Autodesk Inventor part; units mm, degrees
(part 2 of 2)
sketch "Sketch47" plane through (0, 0, 0) normal (0, 0, -1) x (-1, 0, 0)
  arc A0 (-24.47, 4.531) -> (-25.255, 6.4154) centre (-25.8772, 5.0505) ccw projected
  arc A1 (-27.3913, -0.5289) -> (-24.47, 4.531) centre (-29.4449, 4.03) ccw projected
  arc A2 (-29.4158, -0.7913) -> (-27.3913, -0.5289) centre (-28.5449, 0.43) ccw projected
  arc A3 (-29.4158, -0.7913) -> (-29.4739, -0.7913) centre (-29.4449, -0.832) ccw projected
  arc A4 (-31.4984, -0.5289) -> (-29.4739, -0.7913) centre (-30.3449, 0.43) ccw projected
  arc A5 (-34.4197, 4.531) -> (-31.4984, -0.5289) centre (-29.4449, 4.03) ccw projected
  arc A6 (-33.6347, 6.4154) -> (-34.4197, 4.531) centre (-33.0126, 5.0505) ccw projected
  arc A7 (-33.6347, 6.4154) -> (-33.6057, 6.4657) centre (-33.6554, 6.4609) ccw projected
  arc A8 (-32.3662, 8.0878) -> (-33.6057, 6.4657) centre (-32.1126, 6.6094) ccw projected
  arc A9 (-26.5236, 8.0878) -> (-32.3662, 8.0878) centre (-29.4449, 4.03) ccw projected
  arc A10 (-25.2841, 6.4657) -> (-26.5236, 8.0878) centre (-26.7772, 6.6094) ccw projected
  arc A11 (-25.2841, 6.4657) -> (-25.255, 6.4154) centre (-25.2343, 6.4609) ccw projected
  arc A12 (29.4739, -0.7913) -> (31.4984, -0.5289) centre (30.3449, 0.43) ccw projected
  arc A13 (29.4739, -0.7913) -> (29.4158, -0.7913) centre (29.4449, -0.832) ccw projected
  arc A14 (27.3913, -0.5289) -> (29.4158, -0.7913) centre (28.5449, 0.43) ccw projected
  arc A15 (24.47, 4.531) -> (27.3913, -0.5289) centre (29.4449, 4.03) ccw projected
  arc A16 (25.255, 6.4154) -> (24.47, 4.531) centre (25.8772, 5.0505) ccw projected
  arc A17 (25.255, 6.4154) -> (25.2841, 6.4657) centre (25.2343, 6.4609) ccw projected
  arc A18 (26.5236, 8.0878) -> (25.2841, 6.4657) centre (26.7772, 6.6094) ccw projected
  arc A19 (32.3662, 8.0878) -> (26.5236, 8.0878) centre (29.4449, 4.03) ccw projected
  arc A20 (33.6057, 6.4657) -> (32.3662, 8.0878) centre (32.1126, 6.6094) ccw projected
  arc A21 (33.6057, 6.4657) -> (33.6347, 6.4154) centre (33.6554, 6.4609) ccw projected
  arc A22 (34.4197, 4.531) -> (33.6347, 6.4154) centre (33.0126, 5.0505) ccw projected
  arc A23 (31.4984, -0.5289) -> (34.4197, 4.531) centre (29.4449, 4.03) ccw projected
  arc A24 (25.2841, -32.4058) -> (26.5236, -34.0279) centre (26.7772, -32.5495) ccw projected
  arc A25 (25.2841, -32.4058) -> (25.255, -32.3555) centre (25.2343, -32.401) ccw projected
  arc A26 (24.47, -30.4711) -> (25.255, -32.3555) centre (25.8772, -30.9906) ccw projected
  arc A27 (27.3913, -25.4112) -> (24.47, -30.4711) centre (29.4449, -29.97) ccw projected
  arc A28 (29.4158, -25.1488) -> (27.3913, -25.4112) centre (28.5449, -26.37) ccw projected
  arc A29 (29.4158, -25.1488) -> (29.4739, -25.1488) centre (29.4449, -25.1081) ccw projected
  arc A30 (31.4984, -25.4112) -> (29.4739, -25.1488) centre (30.3449, -26.37) ccw projected
  arc A31 (34.4197, -30.4711) -> (31.4984, -25.4112) centre (29.4449, -29.97) ccw projected
  arc A32 (33.6347, -32.3555) -> (34.4197, -30.4711) centre (33.0126, -30.9906) ccw projected
  arc A33 (33.6347, -32.3555) -> (33.6057, -32.4058) centre (33.6554, -32.401) ccw projected
  arc A34 (32.3662, -34.0279) -> (33.6057, -32.4058) centre (32.1126, -32.5495) ccw projected
  arc A35 (26.5236, -34.0279) -> (32.3662, -34.0279) centre (29.4449, -29.97) ccw projected
  arc A36 (-11.2583, -6.47) -> (-8.6603, -7.97) centre (-8.6603, -4.97) ccw projected
  line L0 (-11.2583, -6.47) -> (-15.6081, 1.0639) projected
  arc A37 (-15.6081, 1.0639) -> (-20.4883, 4.5367) centre (-21.3982, -1.9073) ccw projected
  arc A38 (-22.8817, 6.4641) -> (-20.4883, 4.5367) centre (-20.0689, 7.5073) ccw projected
  arc A39 (-22.8817, 6.4641) -> (-23.5653, 7.8287) centre (-29.4449, 4.03) ccw projected
  arc A40 (-22.5454, 12.0548) -> (-23.5653, 7.8287) centre (-21.0454, 9.4567) ccw projected
  line L1 (-22.5454, 12.0548) -> (-10.3994, 19.0673) projected
  arc A41 (-6.2296, 17.8374) -> (-10.3994, 19.0673) centre (-8.8994, 16.4692) ccw projected
  arc A42 (-6.2296, 17.8374) -> (-5.3856, 16.5583) centre (0, 21.03) ccw projected
  arc A43 (-4.9109, 13.5211) -> (-5.3856, 16.5583) centre (-7.6937, 14.6419) ccw projected
  arc A44 (-4.9109, 13.5211) -> (-4.4941, 7.8139) centre (1.1185, 11.0927) ccw projected
  line L2 (-4.4941, 7.8139) -> (0.2887, -0.47) projected
  arc A45 (-4.0415, -7.97) -> (0.2887, -0.47) centre (-4.0415, -2.97) ccw projected
  line L3 (-4.0415, -7.97) -> (-8.6603, -7.97) projected
  line L4 (8.9748, -38.4253) -> (8.0248, -40.0706) projected
  arc A46 (3.7987, -41.0905) -> (8.0248, -40.0706) centre (5.4268, -38.5706) ccw projected
  arc A47 (3.7987, -41.0905) -> (0.7829, -40.014) centre (0, -46.97) ccw projected
  arc A48 (-1.4796, -35.5328) -> (0.7829, -40.014) centre (1.1185, -37.0328) ccw projected
  line L5 (-1.4796, -35.5328) -> (5.4642, -23.5057) projected
  arc A49 (12.4713, -23.6489) -> (5.4642, -23.5057) centre (8.9283, -25.5057) ccw projected
  arc A50 (12.4713, -23.6489) -> (15.6795, -27.0233) centre (20, -19.7033) ccw projected
  arc A51 (14.507, -34.3744) -> (15.6795, -27.0233) centre (13.6463, -30.4681) ccw projected
  arc A52 (14.507, -34.3744) -> (8.9748, -38.4253) centre (16.336, -42.6753) ccw projected
  arc A53 (-25.9281, -2.0225) -> (-23.8122, -0.1261) centre (-29.4449, 4.03) ccw projected
  arc A54 (-18.8001, -0.4073) -> (-23.8122, -0.1261) centre (-21.3982, -1.9073) ccw projected
  line L6 (-18.8001, -0.4073) -> (-15.1554, -6.72) projected
  arc A55 (-17.7535, -11.22) -> (-15.1554, -6.72) centre (-17.7535, -8.22) ccw projected
  line L7 (-17.7535, -11.22) -> (-20.7176, -11.22) projected
  arc A56 (-23.3157, -9.72) -> (-20.7176, -11.22) centre (-20.7176, -8.22) ccw projected
  arc A57 (-23.3157, -9.72) -> (-25.8495, -7.2544) centre (-28.9449, -12.97) ccw projected
  arc A58 (-25.9281, -2.0225) -> (-25.8495, -7.2544) centre (-24.4209, -4.6164) ccw projected
  arc A59 (-20.7176, -14.72) -> (-23.3157, -16.22) centre (-20.7176, -17.72) ccw projected
  line L8 (-20.7176, -14.72) -> (-17.7535, -14.72) projected
  arc A60 (-15.1554, -19.22) -> (-17.7535, -14.72) centre (-17.7535, -17.72) ccw projected
  line L9 (-15.1554, -19.22) -> (-18.8001, -25.5328) projected
  arc A61 (-23.8122, -25.814) -> (-18.8001, -25.5328) centre (-21.3982, -24.0328) ccw projected
  arc A62 (-23.8122, -25.814) -> (-25.9281, -23.9176) centre (-29.4449, -29.97) ccw projected
  arc A63 (-25.8495, -18.6857) -> (-25.9281, -23.9176) centre (-24.4209, -21.3237) ccw projected
  arc A64 (-25.8495, -18.6857) -> (-23.3157, -16.22) centre (-28.9449, -12.97) ccw projected
  arc A65 (15.6795, 1.0833) -> (14.507, 8.4344) centre (13.6463, 4.5281) ccw projected
  arc A66 (15.6795, 1.0833) -> (12.4713, -2.2911) centre (20, -6.2367) ccw projected
  arc A67 (5.4642, -2.4343) -> (12.4713, -2.2911) centre (8.9283, -0.4343) ccw projected
  line L10 (5.4642, -2.4343) -> (-1.4796, 9.5927) projected
  arc A68 (0.7829, 14.0739) -> (-1.4796, 9.5927) centre (1.1185, 11.0927) ccw projected
  arc A69 (0.7829, 14.0739) -> (3.7987, 15.1504) centre (0, 21.03) ccw projected
  arc A70 (8.0248, 14.1305) -> (3.7987, 15.1504) centre (5.4268, 12.6305) ccw projected
  line L11 (8.0248, 14.1305) -> (8.9747, 12.4853) projected
  arc A71 (8.9747, 12.4853) -> (14.507, 8.4344) centre (16.336, 16.7353) ccw projected
  arc A72 (23.6453, -24.7033) -> (28.6453, -19.7033) centre (23.6453, -19.7033) ccw projected
  line L12 (23.6453, -24.7033) -> (20, -24.7033) projected
  arc A73 (15, -19.7033) -> (20, -24.7033) centre (20, -19.7033) ccw projected
  line L13 (15, -19.7033) -> (15, -6.2367) projected
  arc A74 (20, -1.2367) -> (15, -6.2367) centre (20, -6.2367) ccw projected
  line L14 (20, -1.2367) -> (23.6453, -1.2367) projected
  arc A75 (28.6453, -6.2367) -> (23.6453, -1.2367) centre (23.6453, -6.2367) ccw projected
  line L15 (28.6453, -6.2367) -> (28.6453, -19.7033) projected
  arc A76 (0.2887, -25.47) -> (-4.0415, -17.97) centre (-4.0415, -22.97) ccw projected
  line L16 (0.2887, -25.47) -> (-4.5273, -33.8116) projected
  arc A77 (-4.5273, -33.8116) -> (-4.9109, -39.4612) centre (1.1185, -37.0328) ccw projected
  arc A78 (-5.3856, -42.4984) -> (-4.9109, -39.4612) centre (-7.6937, -40.582) ccw projected
  arc A79 (-5.3856, -42.4984) -> (-6.2296, -43.7775) centre (0, -46.97) ccw projected
  arc A80 (-10.3994, -45.0074) -> (-6.2296, -43.7775) centre (-8.8994, -42.4093) ccw projected
  line L17 (-10.3994, -45.0074) -> (-22.5454, -37.9949) projected
  arc A81 (-23.5653, -33.7688) -> (-22.5454, -37.9949) centre (-21.0454, -35.3968) ccw projected
  arc A82 (-23.5653, -33.7688) -> (-22.8817, -32.4042) centre (-29.4449, -29.97) ccw projected
  arc A83 (-20.4883, -30.4768) -> (-22.8817, -32.4042) centre (-20.0689, -33.4474) ccw projected
  arc A84 (-20.4883, -30.4768) -> (-15.93, -27.5616) centre (-21.3982, -24.0328) ccw projected
  line L18 (-15.93, -27.5616) -> (-11.2583, -19.47) projected
  arc A85 (-8.6603, -17.97) -> (-11.2583, -19.47) centre (-8.6603, -20.97) ccw projected
  line L19 (-8.6603, -17.97) -> (-4.0415, -17.97) projected
  circle A86 centre (0, -12.97) radius 4.1 projected
  circle A87 centre (-10, -12.97) radius 1.5 projected
  circle A88 centre (10, -12.97) radius 1.5 projected
  circle A89 centre (31.6453, -19.9117) radius 1.2 projected
  circle A90 centre (31.6453, -6.0284) radius 1.2 projected
  arc A91 (-3.5, -53.0322) -> (6.0622, -50.47) centre (0, -46.97) ccw projected
  line L20 (6.0622, -50.47) -> (12.0059, -40.1753) projected
  arc A92 (16.1615, -37.6783) -> (12.0059, -40.1753) centre (16.336, -42.6753) ccw projected
  line L21 (16.1615, -37.6783) -> (29.6554, -37.2071) projected
  arc A93 (29.6554, -37.2071) -> (31.3743, -36.939) centre (29.4445, -30.2102) ccw projected
  ellipse E0 centre (29.4445, -30.2102) end of major axis (22.4434, -30.2102) minor radius 7 (31.3743, -36.939) -> (36.4456, -30.2102) ccw projected
  line L22 (36.4456, -30.2102) -> (36.4456, 4.2702) projected
  ellipse E1 centre (29.4445, 4.2702) end of major axis (36.4456, 4.2702) minor radius 7 (36.4456, 4.2702) -> (31.374, 10.9991) ccw projected
  arc A94 (31.374, 10.9991) -> (29.6554, 11.2671) centre (29.4445, 4.2702) ccw projected
  line L23 (29.6554, 11.2671) -> (16.1615, 11.7383) projected
  arc A95 (12.0058, 14.2353) -> (16.1615, 11.7383) centre (16.336, 16.7353) ccw projected
  line L24 (12.0058, 14.2353) -> (6.0622, 24.53) projected
  arc A96 (6.0622, 24.53) -> (-3.5, 27.0921) centre (0, 21.03) ccw projected
  line L25 (-32.9449, 10.0921) -> (-3.5, 27.0921) projected
  arc A97 (-32.9449, 10.0921) -> (-36.4449, 4.03) centre (-29.4449, 4.03) ccw projected
  line L26 (-36.4449, -2.97) -> (-36.4449, 4.03) projected
  line L27 (-36.4449, -2.97) -> (-33.4449, -2.97) projected
  arc A98 (-29.4449, -6.97) -> (-33.4449, -2.97) centre (-33.4449, -6.97) ccw projected
  line L28 (-29.4449, -6.97) -> (-29.4449, -9.97) projected
  line L29 (-29.4449, -9.97) -> (-28.9449, -9.97) projected
  arc A99 (-28.9449, -15.97) -> (-28.9449, -9.97) centre (-28.9449, -12.97) ccw projected
  line L30 (-28.9449, -15.97) -> (-29.4449, -15.97) projected
  line L31 (-29.4449, -15.97) -> (-29.4449, -18.97) projected
  arc A100 (-33.4449, -22.97) -> (-29.4449, -18.97) centre (-33.4449, -18.97) ccw projected
  line L32 (-33.4449, -22.97) -> (-36.4449, -22.97) projected
  line L33 (-36.4449, -29.97) -> (-36.4449, -22.97) projected
  arc A101 (-36.4449, -29.97) -> (-32.9449, -36.0322) centre (-29.4449, -29.97) ccw projected
  line L34 (-3.5, -53.0322) -> (-32.9449, -36.0322) projected
  arc A102 (-4.1898, -44.5846) -> (-4.9748, -46.469) centre (-3.5677, -45.9495) ccw projected
  arc A103 (-4.1898, -44.5846) -> (-4.1608, -44.5343) centre (-4.2106, -44.5391) ccw projected
  arc A104 (-2.9213, -42.9122) -> (-4.1608, -44.5343) centre (-2.6677, -44.3906) ccw projected
  arc A105 (2.9213, -42.9122) -> (-2.9213, -42.9122) centre (0, -46.97) ccw projected
  arc A106 (4.1608, -44.5343) -> (2.9213, -42.9122) centre (2.6677, -44.3906) ccw projected
  arc A107 (4.1608, -44.5343) -> (4.1898, -44.5846) centre (4.2106, -44.5391) ccw projected
  arc A108 (4.9748, -46.469) -> (4.1898, -44.5846) centre (3.5677, -45.9495) ccw projected
  arc A109 (2.0535, -51.5289) -> (4.9748, -46.469) centre (0, -46.97) ccw projected
  arc A110 (0.029, -51.7913) -> (2.0535, -51.5289) centre (0.9, -50.57) ccw projected
  arc A111 (0.029, -51.7913) -> (-0.029, -51.7913) centre (0, -51.832) ccw projected
  arc A112 (-2.0535, -51.5289) -> (-0.029, -51.7913) centre (-0.9, -50.57) ccw projected
  arc A113 (-4.9748, -46.469) -> (-2.0535, -51.5289) centre (0, -46.97) ccw projected
  arc A114 (2.9213, 16.9721) -> (4.1608, 18.5942) centre (2.6677, 18.4505) ccw projected
  arc A115 (-2.9213, 16.9721) -> (2.9213, 16.9721) centre (0, 21.03) ccw projected
  arc A116 (-4.1608, 18.5942) -> (-2.9213, 16.9721) centre (-2.6677, 18.4505) ccw projected
  arc A117 (-4.1608, 18.5942) -> (-4.1898, 18.6445) centre (-4.2106, 18.599) ccw projected
  arc A118 (-4.9748, 20.5289) -> (-4.1898, 18.6445) centre (-3.5677, 20.0094) ccw projected
  arc A119 (-2.0535, 25.5888) -> (-4.9748, 20.5289) centre (0, 21.03) ccw projected
  arc A120 (-0.029, 25.8512) -> (-2.0535, 25.5888) centre (-0.9, 24.63) ccw projected
  arc A121 (-0.029, 25.8512) -> (0.029, 25.8512) centre (0, 25.8919) ccw projected
  arc A122 (2.0535, 25.5888) -> (0.029, 25.8512) centre (0.9, 24.63) ccw projected
  arc A123 (4.9748, 20.5289) -> (2.0535, 25.5888) centre (0, 21.03) ccw projected
  arc A124 (4.1898, 18.6445) -> (4.9748, 20.5289) centre (3.5677, 20.0094) ccw projected
  arc A125 (4.1898, 18.6445) -> (4.1608, 18.5942) centre (4.2106, 18.599) ccw projected
  arc A126 (-27.3913, -25.4112) -> (-29.4158, -25.1488) centre (-28.5449, -26.37) ccw projected
  arc A127 (-24.47, -30.4711) -> (-27.3913, -25.4112) centre (-29.4449, -29.97) ccw projected
  arc A128 (-25.255, -32.3555) -> (-24.47, -30.4711) centre (-25.8772, -30.9906) ccw projected
  arc A129 (-25.255, -32.3555) -> (-25.2841, -32.4058) centre (-25.2343, -32.401) ccw projected
  arc A130 (-26.5236, -34.0279) -> (-25.2841, -32.4058) centre (-26.7772, -32.5495) ccw projected
  arc A131 (-32.3662, -34.0279) -> (-26.5236, -34.0279) centre (-29.4449, -29.97) ccw projected
  arc A132 (-33.6057, -32.4058) -> (-32.3662, -34.0279) centre (-32.1126, -32.5495) ccw projected
  arc A133 (-33.6057, -32.4058) -> (-33.6347, -32.3555) centre (-33.6554, -32.401) ccw projected
  arc A134 (-34.4197, -30.4711) -> (-33.6347, -32.3555) centre (-33.0126, -30.9906) ccw projected
  arc A135 (-31.4984, -25.4112) -> (-34.4197, -30.4711) centre (-29.4449, -29.97) ccw projected
  arc A136 (-29.4739, -25.1488) -> (-31.4984, -25.4112) centre (-30.3449, -26.37) ccw projected
  arc A137 (-29.4739, -25.1488) -> (-29.4158, -25.1488) centre (-29.4449, -25.1081) ccw projected
  circle A138 centre (0, -46.97) radius 5
  point P0 (0, 0)
  constraints: 1 centre point, 1 coincident, 2 other
body "Solid1"
